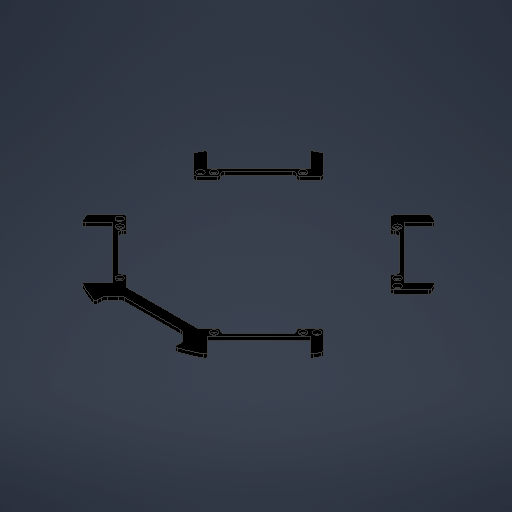
# Autodesk Inventor part: Ground Cover
Saved by Autodesk Inventor 2026.1 (Build 301233020, 233B)
## iProperties
Created: 2026-03-10
Part Number: Ground Cover
Material: Generic
Document SubType Name: Modeling
Designer: Bahaa
Density: 1 g/cm^3
Appearance: Default
Author: Bahaa
Autodesk Inventor part; units mm, degrees
ref_plane "YZ Plane" through (0, 0, 0) normal (1, 0, 0) x (0, 1, 0)
ref_plane "XZ Plane" through (0, 0, 0) normal (0, 1, 0) x (-1, 0, 0)
ref_plane "Work Plane1" through (0, 0, 0) normal (0, 0, 1) x (1, 0, 0)
sketch "Sketch1" plane through (0, 0, 0) normal (0, 0, 1) x (1, 0, 0)
  circle A0 centre (-81.3173, -35.7493) radius 2.85 projected
  circle A1 centre (-81.3173, 30.7188) radius 2.85 projected
  arc A2 (-81.5294, -41.6183) -> (-81.388, -41.3354) centre (-81.883, -41.2647) ccw projected
  line L0 (-81.388, -41.3354) -> (-77.1454, -37.0928) projected
  arc A3 (-77.1454, -37.0928) -> (-77.1454, -34.2643) centre (-78.5596, -35.6786) ccw projected
  line L1 (-79.9031, -31.5066) -> (-77.1454, -34.2643) projected
  arc A4 (-79.9031, -31.5066) -> (-82.7315, -31.5066) centre (-81.3173, -32.9208) ccw projected
  line L2 (-89.7439, -38.5191) -> (-82.7315, -31.5066) projected
  arc A5 (-93.0281, -37.8144) -> (-89.7439, -38.5191) centre (-91.1582, -37.1049) ccw projected
  arc A6 (-93.0281, 32.7839) -> (-93.0281, -37.8144) centre (0, -2.5152) ccw projected
  arc A7 (-89.7439, 33.4886) -> (-93.0281, 32.7839) centre (-91.1582, 32.0744) ccw projected
  line L3 (-82.7315, 26.4761) -> (-89.7439, 33.4886) projected
  arc A8 (-82.7315, 26.4761) -> (-79.9031, 26.4761) centre (-81.3173, 27.8903) ccw projected
  line L4 (-77.1454, 29.2338) -> (-79.9031, 26.4761) projected
  arc A9 (-77.1454, 29.2338) -> (-77.1454, 32.0623) centre (-78.5596, 30.6481) ccw projected
  line L5 (-77.1454, 32.0623) -> (-81.388, 36.3049) projected
  arc A10 (-81.388, 36.3049) -> (-81.5294, 36.5878) centre (-81.883, 36.2342) ccw projected
  line L6 (-92.7805, 47.8388) -> (-81.5294, 36.5878) projected
  arc A11 (-92.7805, 47.8388) -> (-95.1691, 47.4757) centre (-93.8411, 46.7782) ccw projected
  arc A12 (-95.1691, 47.4757) -> (-95.1691, -52.5062) centre (0, -2.5152) ccw projected
  arc A13 (-95.1691, -52.5062) -> (-92.7805, -52.8693) centre (-93.8411, -51.8087) ccw projected
  line L7 (-81.5294, -41.6183) -> (-92.7805, -52.8693) projected
  arc A14 (-43.1335, 70.3168) -> (-43.1335, 71.731) centre (-43.8406, 71.0239) ccw projected
  line L8 (-43.1335, 71.731) -> (-43.8406, 72.4381) projected
  arc A15 (-43.8406, 72.4381) -> (-45.2548, 72.4381) centre (-44.5477, 71.731) ccw projected
  line L9 (-74.9533, 42.7396) -> (-45.2548, 72.4381) projected
  arc A16 (-74.9533, 42.7396) -> (-74.9533, 41.3254) centre (-74.2462, 42.0325) ccw projected
  line L10 (-74.9533, 41.3254) -> (-74.2462, 40.6183) projected
  arc A17 (-74.2462, 40.6183) -> (-72.832, 40.6183) centre (-73.5391, 41.3254) ccw projected
  line L11 (-72.832, 40.6183) -> (-43.1335, 70.3168) projected
  arc A18 (-71.4178, 34.9614) -> (-71.4178, 37.7898) centre (-72.832, 36.3756) ccw projected
  line L12 (-72.1249, 38.4969) -> (-71.4178, 37.7898) projected
  arc A19 (-72.1249, 41.3254) -> (-72.1249, 38.4969) centre (-70.7107, 39.9112) ccw projected
  line L13 (-72.832, 40.6183) -> (-72.1249, 41.3254) projected
  arc A20 (-74.2462, 40.6183) -> (-72.832, 40.6183) centre (-73.5391, 41.3254) ccw projected
  line L14 (-74.9533, 41.3254) -> (-74.2462, 40.6183) projected
  arc A21 (-74.9533, 42.7396) -> (-74.9533, 41.3254) centre (-74.2462, 42.0325) ccw projected
  line L15 (-81.3173, 36.3756) -> (-74.9533, 42.7396) projected
  line L16 (-81.3173, 36.3756) -> (-81.5294, 36.5878) projected
  arc A22 (-81.388, 36.3049) -> (-81.5294, 36.5878) centre (-81.883, 36.2342) ccw projected
  line L17 (-77.1454, 32.0623) -> (-81.388, 36.3049) projected
  arc A23 (-77.1454, 29.2338) -> (-77.1454, 32.0623) centre (-78.5596, 30.6481) ccw projected
  line L18 (-71.4178, 34.9614) -> (-77.1454, 29.2338) projected
  circle A24 centre (-75.6604, 36.3756) radius 1.6 projected
  circle A25 centre (-38.8909, 73.1452) radius 1.6 projected
  line L19 (-45.2548, 72.4381) -> (-38.8909, 78.802) projected
  arc A26 (-43.8406, 72.4381) -> (-45.2548, 72.4381) centre (-44.5477, 71.731) ccw projected
  line L20 (-43.1335, 71.731) -> (-43.8406, 72.4381) projected
  arc A27 (-43.1335, 70.3168) -> (-43.1335, 71.731) centre (-43.8406, 71.0239) ccw projected
  line L21 (-43.8406, 69.6096) -> (-43.1335, 70.3168) projected
  arc A28 (-41.0122, 69.6096) -> (-43.8406, 69.6096) centre (-42.4264, 68.1954) ccw projected
  line L22 (-40.3051, 68.9025) -> (-41.0122, 69.6096) projected
  arc A29 (-40.3051, 68.9025) -> (-37.4767, 68.9025) centre (-38.8909, 70.3168) ccw projected
  line L23 (-31.7491, 74.6301) -> (-37.4767, 68.9025) projected
  arc A30 (-34.5775, 74.6301) -> (-31.7491, 74.6301) centre (-33.1633, 76.0443) ccw projected
  line L24 (-38.8202, 78.8727) -> (-34.5775, 74.6301) projected
  arc A31 (-39.103, 79.0142) -> (-38.8202, 78.8727) centre (-38.7495, 79.3677) ccw projected
  line L25 (-39.103, 79.0142) -> (-38.8909, 78.802) projected
  arc A32 (50.3541, 90.2652) -> (49.991, 92.6538) centre (49.2934, 91.3259) ccw projected
  arc A33 (49.991, 92.6538) -> (-49.991, 92.6538) centre (0, -2.5152) ccw projected
  arc A34 (-49.991, 92.6538) -> (-50.3541, 90.2652) centre (-49.2934, 91.3259) ccw projected
  line L26 (-39.103, 79.0142) -> (-50.3541, 90.2652) projected
  arc A35 (-39.103, 79.0142) -> (-38.8202, 78.8727) centre (-38.7495, 79.3677) ccw projected
  line L27 (-38.8202, 78.8727) -> (-34.5775, 74.6301) projected
  arc A36 (-34.5775, 74.6301) -> (-31.7491, 74.6301) centre (-33.1633, 76.0443) ccw projected
  line L28 (-28.9914, 77.3878) -> (-31.7491, 74.6301) projected
  arc A37 (-28.9914, 77.3878) -> (-28.9914, 80.2162) centre (-30.4056, 78.802) ccw projected
  line L29 (-38.154, 89.3788) -> (-28.9914, 80.2162) projected
  arc A38 (-14, 95.9949) -> (-38.154, 89.3788) centre (0, -2.5152) ccw projected
  line L30 (-14, 95.9949) -> (-14, 76.6241) projected
  arc A39 (-14, 76.6241) -> (-12.8379, 75.6373) centre (-13, 76.6241) ccw projected
  arc A40 (-11.8504, 75.7932) -> (-12.8379, 75.6373) centre (0, -2.5152) ccw projected
  arc A41 (-11.8504, 75.7932) -> (-11, 76.7819) centre (-12, 76.7819) ccw projected
  line L31 (-11, 76.7819) -> (-11, 96.3748) projected
  arc A42 (11, 96.3748) -> (-11, 96.3748) centre (0, -2.5152) ccw projected
  line L32 (11, 96.3748) -> (11, 76.7819) projected
  arc A43 (11, 76.7819) -> (11.8504, 75.7932) centre (12, 76.7819) ccw projected
  arc A44 (12.8379, 75.6373) -> (11.8504, 75.7932) centre (0, -2.5152) ccw projected
  arc A45 (12.8379, 75.6373) -> (14, 76.6241) centre (13, 76.6241) ccw projected
  line L33 (14, 76.6241) -> (14, 95.9949) projected
  arc A46 (38.154, 89.3788) -> (14, 95.9949) centre (0, -2.5152) ccw projected
  line L34 (28.9914, 80.2163) -> (38.154, 89.3788) projected
  arc A47 (28.9914, 80.2163) -> (28.9914, 77.3878) centre (30.4056, 78.802) ccw projected
  line L35 (31.7491, 74.6301) -> (28.9914, 77.3878) projected
  arc A48 (31.7491, 74.6301) -> (34.5775, 74.6301) centre (33.1633, 76.0443) ccw projected
  line L36 (34.5775, 74.6301) -> (38.8202, 78.8727) projected
  arc A49 (38.8202, 78.8727) -> (39.103, 79.0142) centre (38.7494, 79.3677) ccw projected
  line L37 (50.3541, 90.2652) -> (39.103, 79.0142) projected
  circle A50 centre (-36.9121, 94.1788) radius 2.85 projected
  circle A51 centre (38.8909, 73.1452) radius 1.6 projected
  line L38 (38.8909, 78.802) -> (39.103, 79.0142) projected
  arc A52 (38.8202, 78.8727) -> (39.103, 79.0142) centre (38.7494, 79.3677) ccw projected
  line L39 (34.5775, 74.6301) -> (38.8202, 78.8727) projected
  arc A53 (31.7491, 74.6301) -> (34.5775, 74.6301) centre (33.1633, 76.0443) ccw projected
  line L40 (37.4767, 68.9025) -> (31.7491, 74.6301) projected
  arc A54 (37.4767, 68.9025) -> (40.3051, 68.9025) centre (38.8909, 70.3168) ccw projected
  line L41 (41.0122, 69.6096) -> (40.3051, 68.9025) projected
  arc A55 (43.8406, 69.6096) -> (41.0122, 69.6096) centre (42.4264, 68.1954) ccw projected
  line L42 (43.1335, 70.3168) -> (43.8406, 69.6096) projected
  arc A56 (43.1335, 71.731) -> (43.1335, 70.3168) centre (43.8406, 71.0239) ccw projected
  line L43 (43.8406, 72.4381) -> (43.1335, 71.731) projected
  arc A57 (45.2548, 72.4381) -> (43.8406, 72.4381) centre (44.5477, 71.731) ccw projected
  line L44 (38.8909, 78.802) -> (45.2548, 72.4381) projected
  arc A58 (74.9533, 41.3254) -> (74.9533, 42.7396) centre (74.2462, 42.0325) ccw projected
  line L45 (45.2548, 72.4381) -> (74.9533, 42.7396) projected
  arc A59 (45.2548, 72.4381) -> (43.8406, 72.4381) centre (44.5477, 71.731) ccw projected
  line L46 (43.8406, 72.4381) -> (43.1335, 71.731) projected
  arc A60 (43.1335, 71.731) -> (43.1335, 70.3168) centre (43.8406, 71.0239) ccw projected
  line L47 (43.1335, 70.3168) -> (72.832, 40.6183) projected
  arc A61 (72.832, 40.6183) -> (74.2462, 40.6183) centre (73.5391, 41.3254) ccw projected
  line L48 (74.2462, 40.6183) -> (74.9533, 41.3254) projected
  arc A62 (71.4178, 37.7898) -> (71.4178, 34.9614) centre (72.832, 36.3756) ccw projected
  line L49 (77.1454, 29.2338) -> (71.4178, 34.9614) projected
  arc A63 (77.1454, 32.0623) -> (77.1454, 29.2338) centre (78.5596, 30.6481) ccw projected
  line L50 (81.388, 36.3049) -> (77.1454, 32.0623) projected
  arc A64 (81.5294, 36.5878) -> (81.388, 36.3049) centre (81.883, 36.2342) ccw projected
  line L51 (81.5294, 36.5878) -> (81.3173, 36.3756) projected
  line L52 (74.9533, 42.7396) -> (81.3173, 36.3756) projected
  arc A65 (74.9533, 41.3254) -> (74.9533, 42.7396) centre (74.2462, 42.0325) ccw projected
  line L53 (74.2462, 40.6183) -> (74.9533, 41.3254) projected
  arc A66 (72.832, 40.6183) -> (74.2462, 40.6183) centre (73.5391, 41.3254) ccw projected
  line L54 (72.1249, 41.3254) -> (72.832, 40.6183) projected
  arc A67 (72.1249, 38.4969) -> (72.1249, 41.3254) centre (70.7107, 39.9112) ccw projected
  line L55 (71.4178, 37.7898) -> (72.1249, 38.4969) projected
  circle A68 centre (75.6604, 36.3756) radius 1.6 projected
  circle A69 centre (81.3173, -35.7493) radius 2.85 projected
  circle A70 centre (81.3173, 30.7188) radius 2.85 projected
  arc A71 (81.388, -41.3354) -> (81.5294, -41.6182) centre (81.883, -41.2647) ccw projected
  line L56 (92.7805, -52.8693) -> (81.5294, -41.6182) projected
  arc A72 (92.7805, -52.8693) -> (95.1691, -52.5062) centre (93.8411, -51.8087) ccw projected
  arc A73 (95.1691, -52.5062) -> (95.1691, 47.4757) centre (0, -2.5152) ccw projected
  arc A74 (95.1691, 47.4757) -> (92.7805, 47.8388) centre (93.8411, 46.7782) ccw projected
  line L57 (81.5294, 36.5878) -> (92.7805, 47.8388) projected
  arc A75 (81.5294, 36.5878) -> (81.388, 36.3049) centre (81.883, 36.2342) ccw projected
  line L58 (81.388, 36.3049) -> (77.1454, 32.0623) projected
  arc A76 (77.1454, 32.0623) -> (77.1454, 29.2338) centre (78.5596, 30.6481) ccw projected
  line L59 (79.9031, 26.4761) -> (77.1454, 29.2338) projected
  arc A77 (79.9031, 26.4761) -> (82.7315, 26.4761) centre (81.3173, 27.8903) ccw projected
  line L60 (89.7439, 33.4886) -> (82.7315, 26.4761) projected
  arc A78 (93.0281, 32.7839) -> (89.7439, 33.4886) centre (91.1582, 32.0744) ccw projected
  arc A79 (93.0281, -37.8144) -> (93.0281, 32.7839) centre (0, -2.5152) ccw projected
  arc A80 (89.7439, -38.5191) -> (93.0281, -37.8144) centre (91.1582, -37.1049) ccw projected
  line L61 (82.7315, -31.5066) -> (89.7439, -38.5191) projected
  arc A81 (82.7315, -31.5066) -> (79.9031, -31.5066) centre (81.3173, -32.9208) ccw projected
  line L62 (77.1454, -34.2643) -> (79.9031, -31.5066) projected
  arc A82 (77.1454, -34.2643) -> (77.1454, -37.0928) centre (78.5596, -35.6786) ccw projected
  line L63 (77.1454, -37.0928) -> (81.388, -41.3354) projected
  arc A83 (71.4178, -39.9919) -> (71.4178, -42.8203) centre (72.832, -41.4061) ccw projected
  line L64 (72.1249, -43.5274) -> (71.4178, -42.8203) projected
  arc A84 (72.1249, -46.3559) -> (72.1249, -43.5274) centre (70.7107, -44.9417) ccw projected
  line L65 (72.832, -45.6488) -> (72.1249, -46.3559) projected
  arc A85 (74.2462, -45.6488) -> (72.832, -45.6488) centre (73.5391, -46.3559) ccw projected
  line L66 (74.9533, -46.3559) -> (74.2462, -45.6488) projected
  arc A86 (74.9533, -47.7701) -> (74.9533, -46.3559) centre (74.2462, -47.063) ccw projected
  line L67 (81.3173, -41.4061) -> (74.9533, -47.7701) projected
  line L68 (81.3173, -41.4061) -> (81.5294, -41.6182) projected
  arc A87 (81.388, -41.3354) -> (81.5294, -41.6182) centre (81.883, -41.2647) ccw projected
  line L69 (77.1454, -37.0928) -> (81.388, -41.3354) projected
  arc A88 (77.1454, -34.2643) -> (77.1454, -37.0928) centre (78.5596, -35.6786) ccw projected
  line L70 (71.4178, -39.9919) -> (77.1454, -34.2643) projected
  circle A89 centre (75.6604, -41.4061) radius 1.6 projected
  arc A90 (43.8406, -77.4686) -> (45.2548, -77.4686) centre (44.5477, -76.7615) ccw projected
  line L71 (74.9533, -47.7701) -> (45.2548, -77.4686) projected
  arc A91 (74.9533, -47.7701) -> (74.9533, -46.3559) centre (74.2462, -47.063) ccw projected
  line L72 (74.9533, -46.3559) -> (74.2462, -45.6488) projected
  arc A92 (74.2462, -45.6488) -> (72.832, -45.6488) centre (73.5391, -46.3559) ccw projected
  line L73 (72.832, -45.6488) -> (43.1335, -75.3472) projected
  arc A93 (43.1335, -75.3472) -> (43.1335, -76.7615) centre (43.8406, -76.0544) ccw projected
  line L74 (43.1335, -76.7615) -> (43.8406, -77.4686) projected
  circle A94 centre (38.8909, -78.1757) radius 1.6 projected
  line L75 (38.8202, -83.9032) -> (34.5775, -79.6606) projected
  arc A95 (39.103, -84.0447) -> (38.8202, -83.9032) centre (38.7495, -84.3982) ccw projected
  line L76 (39.103, -84.0447) -> (38.8909, -83.8325) projected
  line L77 (45.2548, -77.4686) -> (38.8909, -83.8325) projected
  arc A96 (43.8406, -77.4686) -> (45.2548, -77.4686) centre (44.5477, -76.7615) ccw projected
  line L78 (43.1335, -76.7615) -> (43.8406, -77.4686) projected
  arc A97 (43.1335, -75.3472) -> (43.1335, -76.7615) centre (43.8406, -76.0544) ccw projected
  line L79 (43.8406, -74.6401) -> (43.1335, -75.3472) projected
  arc A98 (41.0122, -74.6401) -> (43.8406, -74.6401) centre (42.4264, -73.2259) ccw projected
  line L80 (40.3051, -73.933) -> (41.0122, -74.6401) projected
  arc A99 (40.3051, -73.933) -> (37.4767, -73.933) centre (38.8909, -75.3472) ccw projected
  line L81 (31.7491, -79.6606) -> (37.4767, -73.933) projected
  arc A100 (34.5775, -79.6606) -> (31.7491, -79.6606) centre (33.1633, -81.0748) ccw projected
  line L82 (-29.4249, -81.9847) -> (29.4249, -81.9847) projected
  line L83 (-31.7491, -79.6606) -> (-29.4249, -81.9847) projected
  arc A101 (-31.7491, -79.6606) -> (-34.5775, -79.6606) centre (-33.1633, -81.0748) ccw projected
  line L84 (-34.5775, -79.6606) -> (-38.8202, -83.9032) projected
  arc A102 (-38.8202, -83.9032) -> (-39.103, -84.0447) centre (-38.7494, -84.3982) ccw projected
  line L85 (-50.3541, -95.2957) -> (-39.103, -84.0447) projected
  arc A103 (-50.3541, -95.2957) -> (-49.991, -97.6843) centre (-49.2934, -96.3564) ccw projected
  arc A104 (-49.991, -97.6843) -> (-34.4811, -104.3352) centre (0, -2.5152) ccw projected
  arc A105 (-34.4811, -104.3352) -> (-32.5, -102.9144) centre (-34, -102.9144) ccw projected
  line L86 (-32.5, -99.5558) -> (-32.5, -102.9144) projected
  arc A106 (-31.0355, -96.0203) -> (-32.5, -99.5558) centre (-27.5, -99.5558) ccw projected
  line L87 (-26.4645, -91.4492) -> (-31.0355, -96.0203) projected
  arc A107 (-22.9289, -89.9847) -> (-26.4645, -91.4492) centre (-22.9289, -94.9847) ccw projected
  line L88 (22.9289, -89.9847) -> (-22.9289, -89.9847) projected
  arc A108 (26.4645, -91.4492) -> (22.9289, -89.9847) centre (22.9289, -94.9847) ccw projected
  line L89 (31.0355, -96.0203) -> (26.4645, -91.4492) projected
  arc A109 (32.5, -99.5558) -> (31.0355, -96.0203) centre (27.5, -99.5558) ccw projected
  line L90 (32.5, -102.9144) -> (32.5, -99.5558) projected
  arc A110 (32.5, -102.9144) -> (34.4811, -104.3352) centre (34, -102.9144) ccw projected
  arc A111 (34.4811, -104.3352) -> (49.991, -97.6843) centre (0, -2.5152) ccw projected
  arc A112 (49.991, -97.6843) -> (50.3541, -95.2957) centre (49.2934, -96.3564) ccw projected
  line L91 (39.103, -84.0447) -> (50.3541, -95.2957) projected
  arc A113 (39.103, -84.0447) -> (38.8202, -83.9032) centre (38.7495, -84.3982) ccw projected
  line L92 (38.8202, -83.9032) -> (34.5775, -79.6606) projected
  arc A114 (34.5775, -79.6606) -> (31.7491, -79.6606) centre (33.1633, -81.0748) ccw projected
  line L93 (29.4249, -81.9847) -> (31.7491, -79.6606) projected
  circle A115 centre (-38.8909, -78.1757) radius 1.6 projected
  line L94 (-38.8909, -83.8325) -> (-39.103, -84.0447) projected
  arc A116 (-38.8202, -83.9032) -> (-39.103, -84.0447) centre (-38.7494, -84.3982) ccw projected
  line L95 (-34.5775, -79.6606) -> (-38.8202, -83.9032) projected
  arc A117 (-31.7491, -79.6606) -> (-34.5775, -79.6606) centre (-33.1633, -81.0748) ccw projected
  line L96 (-37.4767, -73.933) -> (-31.7491, -79.6606) projected
  arc A118 (-37.4767, -73.933) -> (-40.3051, -73.933) centre (-38.8909, -75.3472) ccw projected
  line L97 (-41.0122, -74.6401) -> (-40.3051, -73.933) projected
  arc A119 (-43.8406, -74.6401) -> (-41.0122, -74.6401) centre (-42.4264, -73.2259) ccw projected
  line L98 (-43.1335, -75.3472) -> (-43.8406, -74.6401) projected
  arc A120 (-43.1335, -76.7615) -> (-43.1335, -75.3472) centre (-43.8406, -76.0544) ccw projected
  line L99 (-43.8406, -77.4686) -> (-43.1335, -76.7615) projected
  arc A121 (-45.2548, -77.4686) -> (-43.8406, -77.4686) centre (-44.5477, -76.7615) ccw projected
  line L100 (-38.8909, -83.8325) -> (-45.2548, -77.4686) projected
  arc A122 (-72.832, -45.6488) -> (-74.2462, -45.6488) centre (-73.5391, -46.3559) ccw projected
  line L101 (-74.2462, -45.6488) -> (-74.9533, -46.3559) projected
  arc A123 (-74.9533, -46.3559) -> (-74.9533, -47.7701) centre (-74.2462, -47.063) ccw projected
  line L102 (-45.2548, -77.4686) -> (-74.9533, -47.7701) projected
  arc A124 (-45.2548, -77.4686) -> (-43.8406, -77.4686) centre (-44.5477, -76.7615) ccw projected
  line L103 (-43.8406, -77.4686) -> (-43.1335, -76.7615) projected
  arc A125 (-43.1335, -76.7615) -> (-43.1335, -75.3472) centre (-43.8406, -76.0544) ccw projected
  line L104 (-43.1335, -75.3472) -> (-72.832, -45.6488) projected
  arc A126 (-71.4178, -42.8203) -> (-71.4178, -39.9919) centre (-72.832, -41.4061) ccw projected
  line L105 (-77.1454, -34.2643) -> (-71.4178, -39.9919) projected
  arc A127 (-77.1454, -37.0928) -> (-77.1454, -34.2643) centre (-78.5596, -35.6786) ccw projected
  line L106 (-81.388, -41.3354) -> (-77.1454, -37.0928) projected
  arc A128 (-81.5294, -41.6183) -> (-81.388, -41.3354) centre (-81.883, -41.2647) ccw projected
  line L107 (-81.5294, -41.6183) -> (-81.3173, -41.4061) projected
  line L108 (-74.9533, -47.7701) -> (-81.3173, -41.4061) projected
  arc A129 (-74.9533, -46.3559) -> (-74.9533, -47.7701) centre (-74.2462, -47.063) ccw projected
  line L109 (-74.2462, -45.6488) -> (-74.9533, -46.3559) projected
  arc A130 (-72.832, -45.6488) -> (-74.2462, -45.6488) centre (-73.5391, -46.3559) ccw projected
  line L110 (-72.1249, -46.3559) -> (-72.832, -45.6488) projected
  arc A131 (-72.1249, -43.5274) -> (-72.1249, -46.3559) centre (-70.7107, -44.9417) ccw projected
  line L111 (-71.4178, -42.8203) -> (-72.1249, -43.5274) projected
  circle A132 centre (-75.6604, -41.4061) radius 1.6 projected
  circle A133 centre (0, 0) radius 97.0104
  line L112 (-89.7439, 33.4886) -> (-97.9765, 41.7211)
  line L113 (-89.7439, -38.5191) -> (-97.9765, -46.7516)
  line L114 (-57.9828, 55.4675) -> (-60.1041, 57.5888)
  line L115 (-36.0038, 87.2287) -> (-44.2364, 95.4612)
  line L116 (0, 0) -> (0, 39.9112)
  line L117 (89.7439, 33.4886) -> (97.9765, 41.7211)
  line L118 (36.0038, 87.2287) -> (44.2364, 95.4612)
  line L119 (0, -2.5152) -> (-31.1127, -2.5152)
  line L120 (-89.7439, -38.5191) -> (-97.9765, -46.7516)
  line L121 (-36.0038, -92.2592) -> (-44.2364, -100.4917)
  line L122 (89.7439, -38.5191) -> (97.9765, -46.7516)
  line L123 (36.0038, -92.2592) -> (44.2364, -100.4917)
  line L124 (-60.1041, -62.6193) -> (-57.9828, -60.498)
  line L125 (-36.0038, -92.2592) -> (-27.5772, -83.8325)
  line L126 (-27.5772, -83.8325) -> (-29.4249, -81.9847)
  line L127 (36.0038, -92.2592) -> (27.5772, -83.8325)
  line L128 (27.5772, -83.8325) -> (29.4249, -81.9847)
  point P0 (-90.6924, 34.437)
  point P1 (-90.8389, 34.0487)
  point P2 (90.8389, 34.0487)
  point P3 (90.6924, 34.437)
  constraints: 34 end point, 10 symmetric about line, 4 midpoint, 2 perpendicular, 2 point on circle, 2 point on line, 1 coincident, 1 horizontal, 1 vertical, 3 other
extrude "Extrusion1" add sketch "Sketch1" along normal blind 3 contours L7 A133 L2 A4 L1 A3 L0 A2 | A2 L0 A3 L105 A126 L111 A131 L104 A122 L101 A123 L108 L107 | L7 A13 A12 L113 L2 A133 | A133 L125 L121 A104 A103 L85 | L85 A102 L84 A101 L83 L126 L125 A133 | A123 L101 A122 L104 L124 L102 | L94 L100 A121 L99 A120 L98 A119 L97 A118 L96 A101 L84 A102 | L125 L126 L82 L128 L127 A133 L89 A108 L88 A107 L87 | A133 L87 A106 L86 A105 A104 L121 L125 | L124 L104 L98 A120 L99 A121 L102 | L112 A133 L6 A10 L5 A9 L4 A8 L3 | L112 A12 A11 L6 A133 | A133 L127 L123 A111 A110 L90 A109 L89 | L16 L15 A16 L10 A17 L11 A19 L12 A18 L18 A9 L5 A10 | A133 L29 A37 L28 A30 L24 A31 L26 | L26 A34 A33 L115 L29 A133 | L127 L128 L93 A100 L75 A95 L91 A133 | A133 L91 A112 A111 L123 L127 | A31 L24 A30 L23 A29 L22 A28 L11 A14 L8 A15 L19 L25 | L81 A99 L80 A98 L73 A93 L74 A90 L77 L76 A95 L75 A100 | L9 L114 L11 A17 L10 A16 | A133 L61 L122 A73 A72 L56 | L56 A71 L63 A82 L62 A81 L61 A133 | L9 A15 L8 A14 L11 L114 | L68 L67 A86 L66 A85 L65 A84 L64 A83 L70 A82 L63 A71 | A33 A32 L37 A133 L34 L118 | A133 L37 A49 L36 A48 L35 A47 L34 | A90 L74 A93 L73 L65 A85 L66 A86 L71 | L38 L44 A57 L43 A56 L42 A55 L41 A54 L40 A48 L36 A49 | A133 L117 L60 A77 L59 A63 L50 A64 L57 | L57 A74 A73 L117 A133 | A64 L50 A63 L49 A62 L55 A67 L47 A61 L48 A58 L52 L51 | L45 A58 L48 A61 L47 L42 A56 L43 A57 | A24 | A25 | A51 | A68 | A89 | A94 | A115 | A132
sketch "Sketch2" plane through (0, 0, 3) normal (0, 0, 1) x (1, 0, 0)
  circle A0 centre (75.6604, -41.4061) radius 1.6 projected
  circle A1 centre (38.8909, -78.1757) radius 1.6 projected
  circle A2 centre (-38.8909, -78.1757) radius 1.6
  circle A3 centre (-75.6604, -41.4061) radius 1.6 projected
  circle A4 centre (-75.6604, 36.3756) radius 1.6 projected
  circle A5 centre (-38.8909, 73.1452) radius 1.6 projected
  circle A6 centre (38.8909, 73.1452) radius 1.6 projected
  circle A7 centre (75.6604, 36.3756) radius 1.6 projected
  point P0 (0, 0)
  constraints: 1 centre point, 2 other
hole "Hole1" at (38.8909, -78.1757, 3) at (75.6604, -41.4061, 3) at (-38.8909, -78.1757, 3) at (-75.6604, -41.4061, 3) at (75.6604, 36.3756, 3) at (38.8909, 73.1452, 3) at (-38.8909, 73.1452, 3) at (-75.6604, 36.3756, 3) direction (0, 0, -1) diameter 3.2 end through all counterbore diameter 5.7 counterbore depth 2
fillet "Fillet1" radius 2 6 edges at (-97.9765, 41.7211, 1.5) (-44.2364, 95.4612, 1.5) (44.2364, 95.4612, 1.5) (97.9765, 41.7211, 1.5) (97.9765, -46.7516, 1.5) (-97.9765, -46.7516, 1.5)
body "Solid1"
